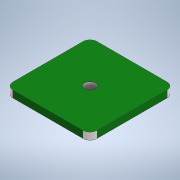
# Autodesk Inventor part: pcbe
Saved by Autodesk Inventor 2022.3 (Build 263350000, 350)
## iProperties
Created: 2022-12-14
Part Number: pcbe
Material: Generic
Document SubType Name: Modeling
Designer: komputer
Density: 1 g/cm^3
Appearance: Default
Author: komputer
Autodesk Inventor part; units mm, degrees
ref_plane "YZ Plane" through (0, 0, 0) normal (1, 0, 0) x (0, 1, 0)
ref_plane "XZ Plane" through (0, 0, 0) normal (0, 1, 0) x (-1, 0, 0)
ref_plane "XY Plane" through (0, 0, 0) normal (0, 0, 1) x (1, 0, 0)
sketch "Sketch1" plane through (0, 0, 0) normal (0, 1, 0) x (-1, 0, 0)
  line L0 (4.1296, 5.0085) -> (-19.8704, 5.0085)
  line L1 (-19.8704, 5.0085) -> (-19.8704, -18.9915)
  line L2 (-19.8704, -18.9915) -> (4.1296, -18.9915)
  line L3 (4.1296, -18.9915) -> (4.1296, 5.0085)
  point P0 (0, 0)
  dimension "d0" = 24
  dimension "d1" = 24
  constraints: 8 end point, 2 parallel, 1 horizontal, 1 perpendicular
  measures "d0" distance of L2.end L1.end
  measures "d1" distance of L1.end L0.end
extrude "Extrusion1" add sketch "Sketch1" along normal blind 2
fillet "Fillet1" radius 2 4 edges at (19.8704, 1, 5.0085) (19.8704, 1, -18.9915) (-4.1296, 1, -18.9915) (-4.1296, 1, 5.0085)
sketch "Sketch2" plane through (0, 2, 0) normal (0, 1, 0) x (1, 0, 0)
  arc A0 (-4.1296, -3.0085) -> (-2.1296, -5.0085) centre (-2.1296, -3.0085) ccw projected
  line L0 (-2.1296, -5.0085) -> (17.8704, -5.0085) projected
  arc A1 (17.8704, -5.0085) -> (19.8704, -3.0085) centre (17.8704, -3.0085) ccw projected
  line L1 (19.8704, -3.0085) -> (19.8704, 16.9915) projected
  arc A2 (19.8704, 16.9915) -> (17.8704, 18.9915) centre (17.8704, 16.9915) ccw projected
  line L2 (17.8704, 18.9915) -> (-2.1296, 18.9915) projected
  arc A3 (-2.1296, 18.9915) -> (-4.1296, 16.9915) centre (-2.1296, 16.9915) ccw projected
  line L3 (-4.1296, 16.9915) -> (-4.1296, -3.0085) projected
  line L4 (-2.1296, -3.0085) -> (17.8704, 16.9915)
  line L5 (17.8704, 16.9915) -> (17.8704, -3.0085)
  line L6 (17.8704, -3.0085) -> (-2.1296, 16.9915)
  circle A4 centre (7.8704, 6.9915) radius 1.5
  point P0 (0, 0)
  dimension "d5" = 3
  constraints: 6 end point, 1 centre point, 1 midpoint, 1 perpendicular, 1 vertical
  measures "d5" diameter of A4
extrude "Extrusion2" cut sketch "Sketch2" against normal blind 2 contours A4 L6 L4 | L4 L6 A4 | L6 A4 L4 | L4 A4 L6
body "Solid1"
